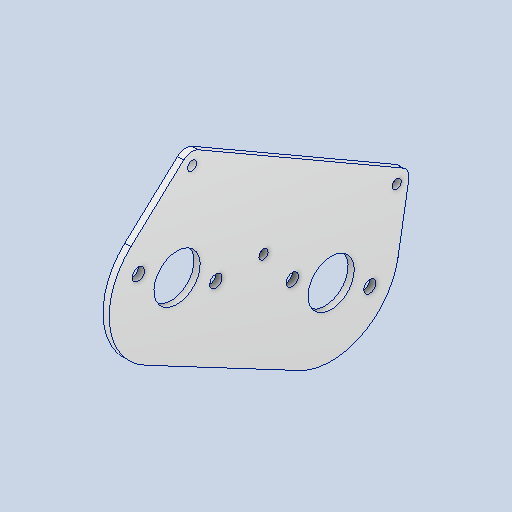
# Autodesk Inventor part: belt_liner_v2_Plate_16
Saved by Autodesk Inventor 2025.2 (Build 292293000, 293)
## iProperties
Created: 2025-01-10
Part Number: belt_liner_v2_Plate_16
Material: アルミニウム 6061
Document SubType Name: Modeling
Designer: haruy
Density: 2.7 g/cm^3
Appearance: アルミニウム - フラット
Author: haruy
Autodesk Inventor part; units mm, degrees
ref_plane "YZ Plane" through (0, 0, 0) normal (1, 0, 0) x (0, 1, 0)
ref_plane "XZ Plane" through (0, 0, 0) normal (0, 1, 0) x (-1, 0, 0)
ref_plane "XY Plane" through (0, 0, 0) normal (0, 0, 1) x (1, 0, 0)
derived "belt_liner_v2_Sketch_Base.ipt"
sketch "スケッチ1" plane through (300, 0, 0) normal (1, 0, 0) x (0, 1, 0)
  circle A0 centre (0, 0) radius 22.36
  circle A1 centre (742.400277, -428.625) radius 23.875 construction
  line L0 (0, 0) -> (0, -985.832038)
  line L1 (4.693429, 56.249257) -> (12.193429, 69.239638)
  line L2 (12.193429, 69.239638) -> (479.847147, -200.760362)
  line L3 (479.847147, -200.760362) -> (472.347147, -213.750743)
  line L4 (472.347147, -213.750743) -> (4.693429, 56.249257)
  line L5 (0, 0) -> (742.400277, -428.625)
  line L6 (-43.599071, -27.395807) -> (-51.099071, -40.386188)
  line L7 (-51.099071, -40.386188) -> (711.003284, -480.386188)
  line L8 (711.003284, -480.386188) -> (718.503284, -467.395807)
  line L9 (718.503284, -467.395807) -> (-43.599071, -27.395807)
  line L10 (-64.855825, 113.724045) -> (-64.855825, 113.724045)
  line L11 (4.693429, 56.249257) -> (0.351336, 58.756166)
  line L12 (0.351336, 58.756166) -> (-2.148664, 54.426038)
  line L13 (-2.148664, 54.426038) -> (2.193429, 51.91913)
  line L14 (2.193429, 51.91913) -> (4.693429, 56.249257)
  line L15 (472.347147, -213.750743) -> (374.172186, -157.069403)
  line L16 (0, -985.832038) -> (0, 0)
  circle A2 centre (0, 0) radius 12.5
  circle A3 centre (0, 0) radius 15
  line L17 (0, 0) -> (0, 0)
  circle A4 centre (0, 0) radius 24.06 construction
  line L18 (0, 0) -> (0, 0)
  line L19 (0, 0) -> (0, 0)
  line L20 (-43.599071, -27.395807) -> (-41.099071, -23.065679)
  line L21 (-41.099071, -23.065679) -> (28.918099, -63.490111)
  line L22 (32.480276, -71.320238) -> (-43.599071, -27.395807)
  line L23 (85.805588, 26.739638) -> (479.847147, -200.760362)
  line L24 (479.847147, -200.760362) -> (482.597147, -195.997222)
  circle A5 centre (742.400277, -428.625) radius 5
  line L25 (718.503284, -467.395807) -> (692.522522, -452.395807)
  line L26 (692.522522, -452.395807) -> (695.022522, -448.065679)
  line L27 (695.022522, -448.065679) -> (721.003284, -463.065679)
  line L28 (721.003284, -463.065679) -> (718.503284, -467.395807)
  circle A6 centre (738.07015, -426.125) radius 5.1
  line L29 (742.400277, -428.625) -> (511.038915, -295.048455)
  circle A7 centre (759.720785, -438.625) radius 5.1
  line L30 (740.62015, -421.70827) -> (762.270785, -434.20827)
  line L31 (735.52015, -430.54173) -> (757.170785, -443.04173)
  circle A8 centre (742.400277, -428.625) radius 22.175 construction
  line L32 (792.376136, -398.519566) -> (776.376136, -426.232379)
  line L33 (776.376136, -426.232379) -> (785.03639, -431.232379)
  line L34 (785.03639, -431.232379) -> (801.03639, -403.519566)
  line L35 (801.03639, -403.519566) -> (792.376136, -398.519566)
  circle A9 centre (738.07015, -426.125) radius 10.1 construction
  circle A10 centre (759.720785, -438.625) radius 10.1 construction
  line L36 (743.12015, -417.378143) -> (764.770785, -429.878143) construction
  line L37 (733.02015, -434.871857) -> (754.670785, -447.371857) construction
  line L38 (743.12015, -417.378143) -> (732.666299, -411.34261) construction
  line L39 (729.323294, -421.075) -> (734.373294, -412.328143) construction
  line L40 (764.770785, -429.878143) -> (773.093818, -434.683448) construction
  line L41 (773.093818, -434.683448) -> (773.43104, -434.878143)
  line L42 (0.351336, 58.756166) -> (-2.148664, 54.426038)
  line L43 (-2.148664, 54.426038) -> (100.487312, -4.83087)
  line L44 (100.487312, -4.83087) -> (102.987312, -0.500743)
  line L45 (102.987312, -0.500743) -> (0.351336, 58.756166)
  line L46 (-51.099071, -40.386188) -> (-51.099071, -619.920903) construction
  line L47 (754.670785, -447.371857) -> (764.770785, -429.878143)
  line L48 (764.770785, -429.878143) -> (773.43104, -434.878143)
  line L49 (773.43104, -434.878143) -> (763.33104, -452.371857)
  line L50 (763.33104, -452.371857) -> (754.670785, -447.371857) construction
  line L51 (479.847147, -200.760362) -> (472.347147, -213.750743)
  line L52 (472.347147, -213.750743) -> (896.699557, -458.750721)
  line L53 (896.699557, -458.750721) -> (904.199557, -445.76034)
  line L54 (904.199557, -445.76034) -> (479.847147, -200.760362)
  line L55 (-12.152186, -2.928204) -> (-38.10869, -47.886188)
  line L56 (-12.152186, -2.928204) -> (25.18381, 61.739638)
  circle A11 centre (38.084445, 34.084194) radius 1.5
  circle A12 centre (59.73508, 21.584194) radius 1.5
  circle A13 centre (711.09303, -460.230743) radius 1.5
  circle A14 centre (0, 0) radius 60
  line L57 (54.694812, -84.145807) -> (57.194812, -79.815679)
  line L58 (100.487312, -4.83087) -> (57.194812, -79.815679)
  circle A15 centre (81.385715, 9.084194) radius 1.5
  circle A16 centre (742.400277, -428.625) radius 6 construction
  circle A17 centre (0, 0) radius 24.06 construction
  circle A18 centre (0, 0) radius 24.06
  circle A19 centre (742.400277, -428.625) radius 24.06
  line L59 (754.430277, -407.788429) -> (12.03, 20.836571)
  circle A20 centre (725.859192, -419.075) radius 4
  circle A21 centre (725.859192, -419.075) radius 1.5
  circle A22 centre (742.400277, -428.625) radius 18.525 construction
  circle A23 centre (748.98688, -417.41667) radius 4
  line L60 (737.43688, -437.421857) -> (742.48688, -428.675)
  circle A24 centre (748.98688, -417.41667) radius 1.5
  line L61 (734.373294, -412.328143) -> (737.823294, -406.352568) construction
  line L62 (737.823294, -406.352568) -> (776.88104, -428.902568)
  line L63 (773.43104, -434.878143) -> (776.88104, -428.902568)
  line L64 (737.823294, -406.352568) -> (723.650341, -415.740187)
  line L65 (720.823294, -435.797432) -> (759.88104, -458.347432)
  line L66 (720.823294, -435.797432) -> (721.866734, -418.829485)
  line L67 (763.33104, -452.371857) -> (759.88104, -458.347432)
  circle A25 centre (735.98688, -439.93333) radius 4
  circle A26 centre (735.98688, -439.93333) radius 1.5
  circle A27 centre (300.529907, 58.653068) radius 120
  line L68 (24.788304, 15.779962) -> (16.12805, 20.779962) construction
  line L69 (896.699557, -458.750721) -> (870.718795, -443.750721)
  line L70 (870.718795, -443.750721) -> (868.218795, -448.080848)
  line L71 (868.218795, -448.080848) -> (894.199557, -463.080848)
  line L72 (894.199557, -463.080848) -> (896.699557, -458.750721)
  circle A28 centre (886.789303, -455.915785) radius 1.5
  line L73 (100.487312, -4.83087) -> (102.987312, -0.500743)
  line L74 (102.987312, -0.500743) -> (112.946604, -6.250743)
  line L75 (112.946604, -6.250743) -> (110.446604, -10.58087)
  line L76 (110.446604, -10.58087) -> (100.487312, -4.83087)
  circle A29 centre (878.129049, -450.915785) radius 1.5
  circle A30 centre (702.432776, -455.230743) radius 1.5
  line L77 (28.918099, -63.490111) -> (57.194812, -79.815679)
  line L78 (479.847147, -200.760362) -> (482.597147, -195.997222)
  line L79 (121.446604, 8.471689) -> (179.903319, -25.278311)
  line L80 (179.903319, -25.278311) -> (182.403319, -20.948184)
  line L81 (182.403319, -20.948184) -> (123.946604, 12.801816)
  line L82 (123.946604, 12.801816) -> (121.446604, 8.471689)
  circle A31 centre (135.905896, 10.515918) radius 4
  circle A32 centre (135.905896, 10.515918) radius 11
  circle A33 centre (161.886659, -4.484082) radius 4
  circle A34 centre (161.886659, -4.484082) radius 11
  line L83 (131.869998, -4.474463) -> (128.369998, -10.536641)
  line L84 (128.369998, -10.536641) -> (147.422557, -21.536641)
  line L85 (147.422557, -21.536641) -> (150.922557, -15.474463)
  line L86 (150.922557, -15.474463) -> (131.869998, -4.474463)
  line L87 (141.396277, -9.974463) -> (137.896277, -16.036641)
  line L88 (157.85076, -19.474463) -> (154.35076, -25.536641)
  line L89 (154.35076, -25.536641) -> (173.403319, -36.536641)
  line L90 (173.403319, -36.536641) -> (176.903319, -30.474463)
  line L91 (176.903319, -30.474463) -> (157.85076, -19.474463)
  line L92 (167.37704, -24.974463) -> (163.87704, -31.036641)
  line L93 (8.443429, 62.744448) -> (900.449557, -452.255531)
  line L94 (170.403319, -41.732794) -> (167.903319, -46.062921)
  line L95 (111.946604, -7.982794) -> (170.403319, -41.732794)
  line L96 (167.903319, -46.062921) -> (109.446604, -12.312921)
  line L97 (109.446604, -12.312921) -> (111.946604, -7.982794)
  circle A35 centre (117.405896, -21.527022) radius 11
  circle A36 centre (117.405896, -21.527022) radius 4
  circle A37 centre (143.386659, -36.527022) radius 11
  circle A38 centre (143.386659, -36.527022) radius 4
  line L98 (140.932176, -2.778311) -> (147.860379, -6.778311)
  line L99 (147.860379, -6.778311) -> (138.360379, -23.232794)
  line L100 (138.360379, -23.232794) -> (131.432176, -19.232794)
  line L101 (131.432176, -19.232794) -> (140.932176, -2.778311)
  line L102 (166.912938, -17.778311) -> (173.841141, -21.778311)
  line L103 (173.841141, -21.778311) -> (164.341141, -38.232794)
  line L104 (164.341141, -38.232794) -> (157.412938, -34.232794)
  line L105 (157.412938, -34.232794) -> (166.912938, -17.778311)
  line L106 (109.446604, -12.312921) -> (96.946604, -33.963556)
  line L107 (96.946604, -33.963556) -> (105.606858, -38.963556)
  line L108 (105.606858, -38.963556) -> (118.106858, -17.312921)
  line L109 (118.106858, -17.312921) -> (109.446604, -12.312921)
  line L110 (109.446604, -12.312921) -> (144.953646, -32.812921)
  line L111 (144.953646, -32.812921) -> (140.953646, -39.741124)
  line L112 (140.953646, -39.741124) -> (105.446604, -19.241124)
  line L113 (105.446604, -19.241124) -> (109.446604, -12.312921)
  line L114 (128.932176, -23.562921) -> (135.860379, -27.562921)
  line L115 (135.860379, -27.562921) -> (134.360379, -30.160997)
  line L116 (134.360379, -30.160997) -> (127.432176, -26.160997)
  line L117 (127.432176, -26.160997) -> (128.932176, -23.562921)
  circle A39 centre (-7.708055, -45.230743) radius 1.25
  circle A40 centre (13.94258, -57.730743) radius 1.25
  circle A41 centre (35.593215, -70.230743) radius 1.25
  circle A42 centre (300.529907, 58.653068) radius 130
  line L118 (300.529907, 58.653068) -> (196.606858, 118.653068)
  line L119 (300.529907, 58.653068) -> (184.618808, 27.594782)
  line L120 (300.529907, 58.653068) -> (269.471621, 174.564167)
  line L121 (272.471621, 179.760319) -> (181.618808, 22.39863)
  line L122 (181.618808, 22.39863) -> (176.422655, 25.39863)
  line L123 (176.422655, 25.39863) -> (267.275469, 182.760319)
  line L124 (267.275469, 182.760319) -> (272.471621, 179.760319)
  line L125 (300.529907, 58.653068) -> (235.529907, -53.930235)
  line L126 (791.376136, -400.251617) -> (788.876136, -404.581744)
  line L127 (788.876136, -404.581744) -> (847.332851, -438.331744)
  line L128 (847.332851, -438.331744) -> (849.832851, -434.001617)
  line L129 (849.832851, -434.001617) -> (791.376136, -400.251617)
  line L130 (849.832851, -434.001617) -> (847.332851, -438.331744)
  line L131 (847.332851, -438.331744) -> (867.218795, -449.812899)
  line L132 (867.218795, -449.812899) -> (869.718795, -445.482772)
  line L133 (869.718795, -445.482772) -> (849.832851, -434.001617)
  line L134 (737.823294, -406.352568) -> (868.218795, -448.080848)
  circle A43 centre (742.400277, -428.625) radius 34.06
  line L135 (859.244569, -445.208978) -> (862.744569, -439.1468)
  circle A44 centre (742.48688, -428.675) radius 8.5
  line L136 (253.202227, 236.679121) -> (109.446604, -12.312921)
  line L137 (249.398857, -49.908508) -> (244.382754, -58.596654)
  line L138 (244.382754, -58.596654) -> (167.903319, -46.062921)
  line L139 (181.618808, 22.39863) -> (198.870869, -5.107736)
  line L140 (267.275469, 182.760319) -> (268.340368, 184.604779)
  circle A45 centre (127.026731, 8.136752) radius 1.5
  circle A46 centre (176.823192, -20.613248) radius 1.5
  circle A47 centre (115.026731, -12.647857) radius 1.5
  circle A48 centre (164.823192, -41.397857) radius 1.5
  line L141 (176.422655, 25.39863) -> (179.422655, 30.594782)
  line L142 (179.422655, 30.594782) -> (175.092528, 33.094782)
  line L143 (175.092528, 33.094782) -> (172.092528, 27.89863)
  line L144 (172.092528, 27.89863) -> (176.422655, 25.39863)
  line L145 (267.275469, 182.760319) -> (264.275469, 177.564167)
  line L146 (264.275469, 177.564167) -> (259.945342, 180.064167)
  line L147 (259.945342, 180.064167) -> (262.945342, 185.260319)
  line L148 (262.945342, 185.260319) -> (267.275469, 182.760319)
  circle A49 centre (263.610405, 181.412243) radius 1.5
  line L149 (268.340368, 184.604779) -> (262.945342, 185.260319)
  line L150 (262.945342, 185.260319) -> (242.144586, 174.804496)
  circle A50 centre (175.757592, 29.246706) radius 1.5
  line L151 (894.199557, -463.080848) -> (718.503284, -467.395807)
  line L152 (695.022522, -448.065679) -> (722.856178, -416.43267)
  line L153 (870.718795, -443.750721) -> (868.218795, -448.080848)
  line L154 (868.218795, -448.080848) -> (861.290592, -444.080848)
  line L155 (861.290592, -444.080848) -> (863.790592, -439.750721)
  line L156 (863.790592, -439.750721) -> (870.718795, -443.750721)
  line L157 (-33.353881, -27.640997) -> (-48.353881, -27.640997)
  line L158 (-48.353881, -27.640997) -> (-48.353881, -280.140997)
  line L159 (-48.353881, -280.140997) -> (-33.353881, -280.140997)
  line L160 (-33.353881, -280.140997) -> (-33.353881, -27.640997)
  line L161 (331.646119, -265.140997) -> (-48.353881, -265.140997)
  line L162 (-48.353881, -265.140997) -> (-48.353881, -280.140997)
  line L163 (-48.353881, -280.140997) -> (331.646119, -280.140997)
  line L164 (331.646119, -280.140997) -> (331.646119, -265.140997)
  line L165 (-20.788182, -57.886188) -> (-13.288182, -44.895807)
  line L166 (5.19258, -72.886188) -> (12.69258, -59.895807)
  line L167 (-48.353881, -74.640997) -> (-71.353881, -74.640997)
  line L168 (-71.353881, -74.640997) -> (-71.353881, -134.640997)
  line L169 (-71.353881, -134.640997) -> (-48.353881, -134.640997)
  line L170 (-48.353881, -134.640997) -> (-48.353881, -74.640997)
  line L171 (-48.353881, -94.640997) -> (-93.353881, -94.640997)
  line L172 (-93.353881, -94.640997) -> (-93.353881, -114.640997)
  line L173 (-93.353881, -114.640997) -> (-48.353881, -114.640997)
  line L174 (-48.353881, -114.640997) -> (-48.353881, -94.640997)
  line L175 (-33.353881, -74.640997) -> (-48.353881, -74.640997)
  line L176 (-93.353881, -104.640997) -> (-48.353881, -104.640997)
  line L177 (-57.353881, -244.640997) -> (-62.353881, -244.640997)
  line L178 (-62.353881, -244.640997) -> (-62.353881, -254.640997)
  line L179 (-62.353881, -254.640997) -> (-57.353881, -254.640997)
  line L180 (-57.353881, -254.640997) -> (-57.353881, -244.640997)
  line L181 (-48.353881, -236.142687) -> (-53.353881, -236.142687)
  line L182 (-53.353881, -236.142687) -> (-53.353881, -262.050693)
  line L183 (-53.353881, -262.050693) -> (-48.353881, -262.050693)
  line L184 (-48.353881, -262.050693) -> (-48.353881, -236.142687)
  line L185 (-50.853881, -236.142687) -> (-50.853881, -262.050693)
  line L186 (301.646119, -265.140997) -> (301.646119, -280.140997)
  line L187 (331.646119, -280.140997) -> (364.16844, -280.140997)
  line L188 (364.16844, -280.140997) -> (371.66844, -267.150616)
  line L189 (331.646119, -265.140997) -> (338.187678, -265.140997)
  line L190 (338.187678, -265.140997) -> (345.687678, -252.150616)
  line L191 (-62.353881, -249.640997) -> (-57.353881, -249.640997)
  line L192 (-89.353881, 250.218666) -> (-109.353881, 250.218666)
  line L193 (-109.353881, 250.218666) -> (-109.353881, -699.60028)
  line L194 (-109.353881, -699.60028) -> (-89.353881, -699.60028)
  line L195 (-89.353881, -699.60028) -> (-89.353881, 250.218666)
  line L196 (263.610405, 181.412243) -> (-89.353881, 181.412243)
  line L197 (-26.7774, -265.289513) -> (-29.28918, -274.968922)
  line L198 (-29.28918, -274.968922) -> (688.535788, -461.242481)
  line L199 (688.535788, -461.242481) -> (691.047567, -451.563072)
  line L200 (691.047567, -451.563072) -> (-26.7774, -265.289513)
  line L201 (-48.353881, -157.96965) -> (-50.353881, -157.96965)
  line L202 (-50.353881, -157.96965) -> (-50.353881, -198.398984)
  line L203 (-50.353881, -198.398984) -> (-48.353881, -198.398984)
  line L204 (-48.353881, -198.398984) -> (-48.353881, -157.96965)
  line L205 (-48.353881, -162.0415) -> (22.746119, -162.0415)
  line L206 (22.746119, -162.0415) -> (22.746119, -204.0415)
  line L207 (22.746119, -204.0415) -> (-48.353881, -204.0415)
  line L208 (-48.353881, -204.0415) -> (-48.353881, -162.0415)
  line L209 (-48.353881, -165.433743) -> (-51.353881, -165.433743)
  line L210 (-51.353881, -165.433743) -> (-51.353881, -191.433743)
  line L211 (-51.353881, -191.433743) -> (-48.353881, -191.433743)
  line L212 (-48.353881, -191.433743) -> (-48.353881, -165.433743)
  line L213 (-51.353881, -177.494923) -> (-75.653881, -177.494923)
  line L214 (-75.653881, -177.494923) -> (-75.653881, -187.494923)
  line L215 (-75.653881, -187.494923) -> (-51.353881, -187.494923)
  line L216 (-51.353881, -187.494923) -> (-51.353881, -177.494923)
  line L217 (-56.353881, -167.251042) -> (-66.353881, -167.251042)
  line L218 (-66.353881, -167.251042) -> (-66.353881, -197.251042)
  line L219 (-66.353881, -197.251042) -> (-56.353881, -197.251042)
  line L220 (-56.353881, -197.251042) -> (-56.353881, -167.251042)
  line L221 (-66.353881, -156.211182) -> (-72.353881, -156.211182)
  line L222 (-72.353881, -156.211182) -> (-72.353881, -222.344302)
  line L223 (-72.353881, -222.344302) -> (-66.353881, -222.344302)
  line L224 (-66.353881, -222.344302) -> (-66.353881, -156.211182)
  circle A51 centre (986.855039, -337.596932) radius 120
  line L225 (54.694812, -84.145807) -> (57.194812, -79.815679)
  line L226 (57.194812, -79.815679) -> (67.154104, -85.565679)
  line L227 (67.154104, -85.565679) -> (64.654104, -89.895807)
  line L228 (64.654104, -89.895807) -> (54.694812, -84.145807)
  line L229 (-43.599071, -27.395807) -> (2.193429, 51.91913)
  line L230 (-19.452821, 14.426725) -> (142.076282, -78.832146)
  circle A52 centre (74.61885, -7.551639) radius 15 construction
  line L231 (64.654104, -89.895807) -> (112.946604, -6.250743)
  circle A53 centre (74.61885, -7.551639) radius 22
  circle A54 centre (67.149719, -35.573275) radius 5 construction
  circle A55 centre (103.616477, -12.410997) radius 5 construction
  circle A56 centre (65.323977, -78.735552) radius 5 construction
  circle A57 centre (11.759787, -74.072312) radius 15
  circle A58 centre (48.161986, -57.492809) radius 15 construction
  circle A59 centre (48.161986, -57.492809) radius 22
  circle A60 centre (103.616477, -12.410997) radius 3 construction
  circle A61 centre (103.616477, -12.410997) radius 1.5
  circle A62 centre (67.149719, -35.573275) radius 3 construction
  circle A63 centre (67.149719, -35.573275) radius 1.5
  circle A64 centre (65.323977, -78.735552) radius 3 construction
  circle A65 centre (65.323977, -78.735552) radius 1.5
  circle A66 centre (103.616477, -12.410997) radius 4
  circle A67 centre (67.149719, -35.573275) radius 4
  circle A68 centre (65.323977, -78.735552) radius 4
  circle A69 centre (74.61885, -7.551639) radius 7.5
  circle A70 centre (48.161986, -57.492809) radius 7.5
  circle A71 centre (74.61885, -7.551639) radius 14.5
  circle A72 centre (48.161986, -57.492809) radius 14.5
  circle A73 centre (81.86885, 5.00573) radius 2
  circle A74 centre (67.36885, -20.109007) radius 2
  line L232 (81.86885, 5.00573) -> (67.36885, -20.109007)
  circle A75 centre (55.411986, -44.935441) radius 2
  circle A76 centre (40.911986, -70.050177) radius 2
  line L233 (55.411986, -44.935441) -> (40.911986, -70.050177)
  line L234 (106.554342, -9.696416) -> (90.777108, 7.378555)
  line L235 (55.178321, 2.747188) -> (28.721457, -47.193983)
  line L236 (44.405095, -79.169658) -> (64.640906, -82.676798)
  line L237 (68.788079, -80.735552) -> (107.080579, -14.410997)
  circle A77 centre (0, 0) radius 24.06
  line L238 (854.261054, -442.331744) -> (857.761054, -436.269566) construction
  line L239 (861.290592, -444.080848) -> (863.790592, -439.750721)
  line L240 (863.790592, -439.750721) -> (857.728414, -436.250721)
  line L241 (857.728414, -436.250721) -> (855.228414, -440.580848)
  line L242 (855.228414, -440.580848) -> (861.290592, -444.080848)
  line L243 (849.832851, -434.001617) -> (864.427288, -408.723309)
  line L244 (859.332851, -417.547134) -> (861.832851, -413.217007)
  line L245 (861.832851, -413.217007) -> (842.253241, -401.912714)
  line L246 (842.253241, -401.912714) -> (839.753241, -406.242841)
  line L247 (839.753241, -406.242841) -> (859.332851, -417.547134)
  line L248 (913.524875, -454.608416) -> (917.855002, -457.108416)
  line L249 (917.855002, -457.108416) -> (928.855002, -438.055858)
  line L250 (928.855002, -438.055858) -> (924.524875, -435.555858)
  line L251 (924.524875, -435.555858) -> (913.524875, -454.608416)
  line L252 (916.024875, -450.278289) -> (922.024875, -439.885985)
  line L253 (922.024875, -439.885985) -> (909.900519, -432.885985)
  line L254 (909.900519, -432.885985) -> (903.900519, -443.278289)
  line L255 (903.900519, -443.278289) -> (916.024875, -450.278289)
  line L256 (905.400519, -440.680213) -> (908.400519, -435.484061)
  line L257 (908.400519, -435.484061) -> (863.832851, -409.752905)
  line L258 (863.832851, -409.752905) -> (860.832851, -414.949058)
  line L259 (860.832851, -414.949058) -> (905.400519, -440.680213)
  line L260 (878.08963, -417.984061) -> (875.08963, -423.180213)
  line L261 (897.271354, -441.76034) -> (902.900519, -445.01034)
  line L262 (924.524875, -435.555858) -> (907.524875, -465.000721)
  line L263 (907.524875, -465.000721) -> (903.194748, -462.500721)
  line L264 (903.194748, -462.500721) -> (920.194748, -433.055858)
  line L265 (920.194748, -433.055858) -> (924.524875, -435.555858)
  line L266 (896.699557, -458.750721) -> (907.524875, -465.000721)
  line L267 (907.524875, -465.000721) -> (905.024875, -469.330848)
  line L268 (905.024875, -469.330848) -> (894.199557, -463.080848)
  line L269 (894.199557, -463.080848) -> (896.699557, -458.750721)
  point P0 (732.666299, -411.34261)
  point P1 (-0.898664, 56.591102)
  point P2 (-30.60869, -34.895807)
  point P3 (-40.853881, -37.640997)
  point P4 (-40.853881, -272.640997)
  point P5 (321.646119, -272.640997)
  point P6 (311.646119, -272.640997)
  point P7 (351.022615, -263.890997)
  point P8 (359.682869, -268.890997)
  point P9 (-18.353881, -272.640997)
  point P10 (680.112268, -453.890997)
  dimension "d12" = 29
  dimension "d13" = 29
  dimension "d1" = 6
  dimension "d2" = 3
  dimension "d3" = 6
  dimension "d4" = 3
  dimension "d5" = 6
  dimension "d6" = 3
  dimension "d7" = 8
  dimension "d8" = 8
  dimension "d9" = 8
  dimension "d10" = 15
  dimension "d11" = 15
  dimension "d14" = 4
  dimension "d17" = 360
  dimension "d19" = 4
  dimension "d22" = 360
  measures "d1" diameter of A60
  measures "d2" diameter of A61
  measures "d3" diameter of A62
  measures "d4" diameter of A63
  measures "d5" diameter of A64
  measures "d6" diameter of A65
  measures "d7" diameter of A66
  measures "d8" diameter of A67
  measures "d9" diameter of A68
  measures "d10" diameter of A69
  measures "d11" diameter of A70
  measures "d14" diameter of A73
  measures "d19" diameter of A75
extrude "押し出し1" add sketch "スケッチ1" against normal blind 2 contours L235 L59 A53 A14 L230 | L230 A14 L5 L235 | L235 A53 L59 | L5 A14 A59 L235 | L230 A67 L5 A14 | A14 A53 L59 L58 L230 A67 | A53 L4 L43 A73 | L43 A73 A71 L59 A14 A53 | A14 L59 A53 | L59 A14 A53 | L5 A67 L58 A59 A14 | A59 A14 | A14 L59 A71 A74 A53 | A67 L230 A63 | L230 A63 A67 L5 | A53 L4 | L5 A67 | A59 L58 L77 A76 A72 A75 L21 A14 | A53 L58 L59 | L59 A71 A73 L43 A53 L58 | A73 L232 A69 L59 A71 | A53 L234 L4 | L4 L234 L44 L43 A53 | L59 A69 L232 A74 A71 | L21 L77 A76 A59 L9 | A67 L230 L58 L5 | A59 L58 | L58 L5 L237 A68 L236 L226 A59 | L59 L237 L230 L58 | L58 A53 L76 L234 A66 L237 L59 | A71 A74 L232 A69 L59 | L59 A69 L232 A73 A71 | L58 A53 | L43 L58 A53 | L9 A59 | L58 L230 L237 L5 | L58 L77 A59 | L44 L234 L76 | A59 L9 L236 | L226 L236 L57 | L57 L236 L9 A59 L77 | A66 | A72 A75 L233 A70 A76 | A68 | A76 L233 A70 A75 A72 | A15 | A41
